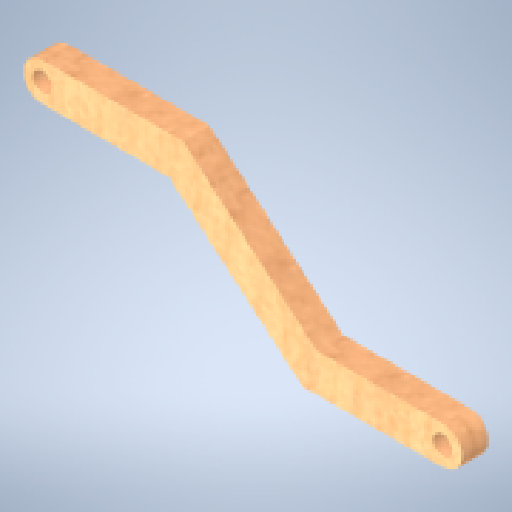
# Autodesk Inventor part: BrazoTV2
Saved by Autodesk Inventor 2023.1 (Build 271208000, 208)
## iProperties
Created: 2022-10-30
Part Number: BrazoTV2
Material: MDF Medium Density Fiberboard
Document SubType Name: Modeling
Designer: Daniel Peña
Density: 0.8 g/cm^3
Appearance: Cherry - Natural Low Gloss
Author: Daniel Peña
Autodesk Inventor part; units mm, degrees
ref_plane "YZ Plane" through (0, 0, 0) normal (1, 0, 0) x (0, 1, 0)
ref_plane "XZ Plane" through (0, 0, 0) normal (0, 1, 0) x (-1, 0, 0)
ref_plane "XY Plane" through (0, 0, 0) normal (0, 0, 1) x (1, 0, 0)
sketch "Sketch1" plane through (0, 0, 0) normal (0, 0, 1) x (1, 0, 0)
  line L0 (-16.7246, 10.0225) -> (18.2754, 10.0225) construction
  line L1 (53.2754, -19.9775) -> (88.2754, -19.9775) construction
  line L2 (18.2754, 10.0225) -> (53.2754, -19.9775) construction
  line L3 (-16.7246, 15.0225) -> (20.125, 15.0225)
  line L4 (20.125, 15.0225) -> (55.125, -14.9775)
  line L5 (55.125, -14.9775) -> (88.2754, -14.9775)
  line L6 (-16.7246, 5.0225) -> (16.4258, 5.0225)
  line L7 (16.4258, 5.0225) -> (51.4258, -24.9775)
  line L8 (51.4258, -24.9775) -> (88.2754, -24.9775)
  line L9 (-21.7246, 10.0225) -> (-21.7246, 10.0225)
  line L10 (93.2754, -19.9775) -> (93.2754, -19.9775)
  arc A0 (-21.7246, 10.0225) -> (-16.7246, 5.0225) centre (-16.7246, 10.0225) ccw
  arc A1 (-16.7246, 15.0225) -> (-21.7246, 10.0225) centre (-16.7246, 10.0225) ccw
  arc A2 (88.2754, -24.9775) -> (93.2754, -19.9775) centre (88.2754, -19.9775) ccw
  arc A3 (93.2754, -19.9775) -> (88.2754, -14.9775) centre (88.2754, -19.9775) ccw
  point P0 (0, 0)
  point P1 (93.2754, -19.9775)
  dimension "d0" = 35
  dimension "d4" = 35
  dimension "d5" = 35
  dimension "d6" = 30
  dimension "d7" = 5
  dimension "d8" = 5
  dimension "d10" = 5
  dimension "d11" = 5
  dimension "d12" = 5
  dimension "d22" = 5
  dimension "d23" = 5
  dimension "d24" = 5
  dimension "d25" = 5
  constraints: 22 end point, 8 point on circle, 8 tangent, 4 centre point, 3 equal radius, 2 vertical, 1 horizontal
  measures "d0" distance of L0.start L0.end
  measures "d4" distance of L1.start L1.end
  measures "d5" horizontal distance of L1.start L0.end
  measures "d6" vertical distance of L1.start L0.end
  measures "d7" distance between parallel lines of L0 L3
  measures "d8" distance between parallel lines of L0 L6
  measures "d10" distance from line of L0.start L9
  measures "d11" distance from line of L10 L1.end
  measures "d12" radius of A0
  measures "d22" distance between parallel lines of L8 L1
  measures "d23" distance between parallel lines of L5 L1
  measures "d24" distance between parallel lines of L4 L2
  measures "d25" distance between parallel lines of L7 L2
extrude "Extrusion1" add sketch "Sketch1" along normal blind 7
sketch "Sketch2" plane through (0, 0, 7) normal (0, 0, 1) x (1, 0, 0)
  arc A0 (-16.7246, 15.0225) -> (-16.7246, 5.0225) centre (-16.7246, 10.0225) ccw projected
  arc A1 (88.2754, -24.9775) -> (88.2754, -14.9775) centre (88.2754, -19.9775) ccw projected
  point P0 (0, 0)
  constraints: 2 coincident
hole "Hole1" at (-16.7246, 10.0225, 7) at (88.2754, -19.9775, 7) direction (0, 0, -1) diameter 5 end through all
body "Solid1"
